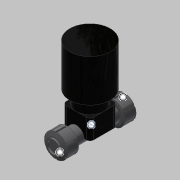
# Autodesk Inventor part: DIAPHRAGM VALVE PNEUMATIC GLUED DN15
Saved by Autodesk Inventor 2017 (Build 210142000, 142)
## iProperties
Created: 2016-04-26
Part Number: DIAPHRAGM VALVE PNEUMATIC GLUED DN15
Description: DKUIV
Document SubType Name: Modeling
Manufacturer: SEKISUI
Mass: 197.859 g
Surface Area: 285.44 cm^2
Volume: 153.379 cm^3
Density: 1.29 g/cm^3
Material: PVC
Appearance: Smooth - White(2)
Catalog Web Link: http://www.pocketbrewery.com
Title: BALL VALVE PVC-U TRD DN15
Autodesk Inventor part; units mm, degrees
ref_plane "YZ Plane" through (0, 0, 0) normal (1, 0, 0) x (0, 1, 0)
ref_plane "XZ Plane" through (0, 0, 0) normal (0, 1, 0) x (-1, 0, 0)
ref_plane "XY Plane" through (0, 0, 0) normal (0, 0, 1) x (1, 0, 0)
sketch "Sketch_1" plane through (0, 0, 0) normal (1, 0, 0) x (0, 1, 0)
  line L0 (61.0702, 0) -> (61.0702, -13.6667)
  line L1 (61.0702, -13.6667) -> (58.5831, -20.5)
  line L2 (58.5831, -20.5) -> (40.0529, -20.5)
  line L3 (40.0529, -20.5) -> (38.848, -17.1896)
  line L4 (38.848, -17.1896) -> (38.848, -13.6667)
  line L5 (-38.848, -13.6667) -> (-38.848, -17.1896)
  line L6 (-38.848, -17.1896) -> (-40.0529, -20.5)
  line L7 (-40.0529, -20.5) -> (-58.5831, -20.5)
  line L8 (-58.5831, -20.5) -> (-61.0702, -13.6667)
  line L9 (-61.0702, -13.6667) -> (-61.0702, 0)
  line L10 (-61.0702, 0) -> (61.0702, 0)
  line L11 (-40.0529, -20.5) -> (0, -20.5) construction
  line L12 (0, -20.5) -> (0, -30.1874) construction
  line L13 (-59.3111, -20.5) -> (-42.0529, -20.5)
  line L14 (-42.0529, -20.5) -> (-42.0529, -18.5)
  line L15 (-42.0529, -18.5) -> (-59.3111, -18.5)
  line L16 (-59.3111, -18.5) -> (-59.3111, -20.5)
  line L17 (42.0529, -20.5) -> (59.3111, -20.5)
  line L18 (59.3111, -20.5) -> (59.3111, -18.5)
  line L19 (59.3111, -18.5) -> (42.0529, -18.5)
  line L20 (42.0529, -18.5) -> (42.0529, -20.5)
  line L21 (-38.848, -13.6667) -> (38.848, -13.6667)
  point P0 (0, 0)
  point P1 (0, 0)
  point P2 (-49.318, -20.5)
  point P3 (50.682, -20.5)
  point P4 (0, 0)
  dimension "dimE" = 41
  dimension "d22" = 20.5
  dimension "d23" = 6.8333
  dimension "d24" = 20
  dimension "d27" = 22.2222
  dimension "d28" = 22.2222
  dimension "d52" = 20
  dimension "d53" = 2
  dimension "d54" = 2
  dimension "d55" = 2
  dimension "dimZ" = 100
  constraints: 44 end point, 6 parallel, 5 equal length, 5 horizontal, 5 perpendicular, 4 point on line, 3 collinear, 3 midpoint, 2 coincident
  measures "dimE" diameter of L2 L10
  measures "d22" distance from line of L0.start L2
  measures "d23" vertical distance of L0.end L1.end
  measures "d24" angle of L0 L1
  measures "d27" distance between parallel lines of L9 L5
  measures "d28" distance between parallel lines of L0 L4
  measures "d52" angle of L5 L6
  measures "d53" distance of L15.end L13.start
  measures "d54" distance from line of L6.end L14
  measures "d55" distance from line of L2.end L20
  measures "dimZ" distance of point (50.682, -20.5) point (-49.318, -20.5)
revolve "Revolution1" add sketch "Sketch_1" angle 360 about axis through (0, -61.0702, 0) along (0, 1, 0) contours L0 L1 L19 L20 L2 L3 L4 L21 L5 L6 L7 L14 L15 L8 L9 L10 | L1 L2 L20 L19 | L15 L14 L7 L8 | L8 L13 L16
sketch "Sketch11" plane through (0, 0, 0) normal (0, 0, 1) x (1, 0, 0)
  line L0 (-23.848, 23.848) -> (23.848, 23.848)
  line L1 (23.848, 23.848) -> (23.848, -23.848)
  line L2 (23.848, -23.848) -> (-23.848, -23.848)
  line L3 (-23.848, -23.848) -> (-23.848, 23.848)
  line L4 (23.848, -23.848) -> (-23.848, 23.848)
  line L5 (17.1896, 38.848) -> (-17.1896, 38.848) projected
  point P0 (0, 0)
  point P1 (0, 0)
  point P2 (0, 0)
  dimension "d71" = 15
  constraints: 10 end point, 2 coincident, 2 parallel, 2 perpendicular, 1 horizontal, 1 midpoint
  measures "d71" distance between parallel lines of L0 L5
extrude "Extrusion6" add sketch "Sketch11" along normal blind 34
sketch "Sketch_2" plane through (0, 0, 0) normal (1, 0, 0) x (0, 1, 0)
  line L0 (0, 34) -> (23.848, 34)
  line L1 (23.848, 34) -> (23.848, 56.2222)
  line L2 (23.848, 56.2222) -> (0, 56.2222)
  line L3 (0, 56.2222) -> (0, 34)
  line L4 (0, 56.2222) -> (34.9591, 56.2222)
  line L5 (34.9591, 56.2222) -> (34.9591, 129)
  line L6 (34.9591, 129) -> (0, 129)
  line L7 (0, 129) -> (0, 56.2222)
  line L8 (-33.3229, 0) -> (54.4515, 0)
  line L9 (-90.3, 0) -> (90.3, 0) projected
  line L10 (0, -319.9275) -> (0, 424.6014) projected
  point P0 (10.5643, 0)
  dimension "d67" = 22.2222
  dimension "d68" = 129
  dimension "d70" = 11.1111
  constraints: 18 end point, 4 parallel, 2 horizontal, 2 perpendicular, 1 coincident, 1 collinear, 1 midpoint, 1 point on line
  measures "d67" distance of L0.end L1.end
  measures "d68" distance between parallel lines of L6 L8
  measures "d70" distance between parallel lines of L5 L1
revolve "Revolution2" add sketch "Sketch_2" angle 360 about axis through (0, 0, 129) along (0, 0, -1)
fillet "Fillet1" radius 6.7 4 edges at (-23.848, 23.848, 17) (-23.848, -23.848, 17) (23.848, -23.848, 17) (23.848, 23.848, 17)
sketch "Sketch_7" plane through (0, 0, 0) normal (1, 0, 0) x (0, 1, 0)
  line L0 (-64.5, 12.5) -> (64.5, 12.5)
  line L1 (48.5126, 0) -> (-48.5126, 0)
  line L2 (-64.5, 12.5) -> (-64.5, 10)
  line L3 (-64.5, 10) -> (64.5, 10)
  line L4 (64.5, 10) -> (64.5, 12.5)
  line L5 (0, 0.4963) -> (0, 17.9963)
  point P0 (0, 0)
  point P1 (0, 0)
  point P2 (0, 10)
  point P3 (0, 0)
  dimension "dimH" = 129
  dimension "dimD" = 20
  dimension "dimD2" = 25
  constraints: 12 end point, 2 coincident, 2 midpoint, 2 perpendicular, 2 point on line, 2 vertical, 1 horizontal, 1 parallel
  measures "dimH" distance of L2.end L3.end
  measures "dimD" diameter of L3 L1
  measures "dimD2" diameter of L0 L1
revolve "Revolution3" add sketch "Sketch_7" angle 360 about axis through (0, 48.5126, 0) along (0, -1, 0)
extrude "Extrusion8" cut sketch "Sketch_1" along normal mid plane 2.7333 contours L18 L17 L1 | L1 L2 L20 L19 | L15 L14 L7 L8 | L8 L13 L16
pattern_circular "Circular Pattern1" count 6 over 360 about axis through (0, 32.25, 0) along (0, -1, 0) of "Extrusion8"
equation "\"d23\" = 0.333333 * d22"
equation "\"d27\" = 0.222222 * dimZ"
equation "\"d28\" = d27"
equation "\"d35\" = 0.1 * dimC"
equation "\"d47\" = 0.0666667 * dimE"
equation "\"dimC\" = 67"
body "Solid1"
